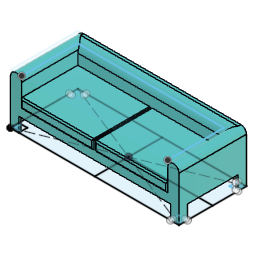
lego_sofa v5 (Autodesk Fusion 360 design; units mm, degrees)
Autodesk Fusion 360 part; units mm, degrees
note: some values were not read from the file. Chosen so that the rebuilt part matches the saved one: which pieces of a blend or face edit are solid.
sketch "Skizze1" plane through (0, 0, 0) normal (0, 0, 1) x (1, 0, 0)
  line L0 (30, -12) -> (-30, -12)
  line L1 (-30, -12) -> (-30, 12)
  line L2 (-30, 12) -> (30, 12)
  line L3 (30, 12) -> (30, -12)
  line L4 (30, -12) -> (-30, 12) construction
  line L5 (-30, -12) -> (30, 12) construction
  dimension "d1" = 60
  dimension "d2" = 24
  constraint horizontal L0
  constraint perpendicular L0 L1
  constraint parallel L0 L2
  constraint parallel L1 L3
  constraint coincident L4 origin
  constraint coincident L5 origin
  measures "d1" distance of L1.end L2.end
  measures "d2" distance of L0.end L1.end
extrude "Extrusion1" add sketch "Skizze1" along normal blind 18
sketch "Skizze2" plane through (0, 0, 0) normal (0, 0, -1) x (1, 0, 0)
  line L0 (-30, -12) -> (30, -12)
  line L1 (30, -12) -> (30, 12)
  line L2 (30, 12) -> (-30, 12)
  line L3 (-30, 12) -> (-30, -12)
  line L4 (-30, 12) -> (-27, 12)
  line L5 (-27, 12) -> (-27, 9)
  line L6 (-27, 9) -> (-30, 9)
  line L7 (-30, 9) -> (-30, 12)
  line L8 (27, 9) -> (30, 9)
  line L9 (27, 12) -> (27, 9)
  line L10 (27, -9) -> (30, -9)
  line L11 (27, -12) -> (27, -9)
  line L12 (-27, -9) -> (-30, -9)
  line L13 (-27, -12) -> (-27, -9)
  line L14 (-29.25, 9.75) -> (-29.25, 11.25)
  line L15 (-29.25, 11.25) -> (-27.75, 11.25)
  line L16 (-29.25, 9.75) -> (-29.25, 9)
  line L17 (-27.75, 11.25) -> (-27, 11.25)
  line L18 (0, 12) -> (0, -12)
  line L19 (0, 0) -> (30, 0)
  line L20 (-29.25, 11.25) -> (-29.25, 9)
  line L21 (-29.25, 11.25) -> (-27, 11.25)
  line L22 (29.25, 11.25) -> (29.25, 9)
  line L23 (29.25, 11.25) -> (27, 11.25)
  line L24 (29.25, -11.25) -> (27, -11.25)
  line L25 (29.25, -11.25) -> (29.25, -9)
  line L26 (-29.25, -11.25) -> (-27, -11.25)
  line L27 (-29.25, -11.25) -> (-29.25, -9)
  dimension "d5" = 3
  dimension "d6" = 3
  constraint horizontal L4
  constraint vertical L5
  constraint horizontal L6
  constraint vertical L7
  constraint coincident L2.end L3.start
  constraint coincident L6 L16.end
  constraint perpendicular L6 L16
  constraint coincident L5 L17.end
  constraint perpendicular L5 L17
  constraint parallel L7 L14
  constraint parallel L4 L15
  constraint midpoint L2 L18.start
  constraint midpoint L0 L18.end
  constraint midpoint L18 L19.start
  constraint midpoint L1 L19.end
  constraint symmetric L14.end L18 L22.start
  constraint symmetric L16.end L18 L22.end
  constraint symmetric L17.end L18 L23.end
  constraint symmetric L19 L22.start L24.start
  constraint symmetric L19 L22.end L25.end
  constraint symmetric L19 L23.end L24.end
  constraint symmetric L18 L24.start L26.start
  constraint symmetric L18 L24.end L26.end
  constraint symmetric L18 L25.end L27.end
  measures "d5" distance of L2.end L4.end
  measures "d6" distance of L2.end L6.end
extrude "Extrusion2" cut sketch "Skizze2" against normal blind 5 contours L0 L2 L3 L5 L6 L12 L13 L18 | L0 L1 L10 L11 L18 L19 | L1 L2 L8 L9 L18 L19
sketch "Skizze3" plane through (0, 0, 18) normal (0, 0, 1) x (-1, 0, 0)
  line L0 (-30, -12) -> (30, -12)
  line L1 (30, -12) -> (30, 12)
  line L2 (30, 12) -> (-30, 12)
  line L3 (-30, 12) -> (-30, -12)
  line L4 (-26, -8) -> (26, -8)
  line L5 (26, -8) -> (26, 8)
  line L6 (-26, 8) -> (-26, -8)
  line L7 (26, 8) -> (26, 12)
  line L8 (-26, 8) -> (-26, 12)
  constraint parallel L0 L4
  constraint parallel L1 L5
  constraint parallel L3 L6
  constraint coincident L2 L7.end
  constraint perpendicular L2 L7
  constraint coincident L2 L8.end
  constraint perpendicular L2 L8
extrude "Extrusion3" cut sketch "Skizze3" against normal blind 7 contours L2 L4 L5 L6 L7 L8
fillet "Abrundung1" radius 3 1 edges at (0, 8, 18)
fillet "Abrundung2" radius 2 4 edges at (30, 0, 18) (26, -0.5, 18) (-26, -0.5, 18) (-30, 0, 18)
extrude "Extrusion4" cut sketch "Skizze2" against normal blind 5 contours L12 L13 L26 L27 | L5 L6 L14 L15 L16 L17 L20 L21 | L10 L11 L24 L25 | L8 L9 L22 L23
sketch "Skizze4" plane through (0, 0, 0) normal (0, 0, -1) x (1, 0, 0)
sketch "Skizze14" plane through (0, 0, 11) normal (0, 0, 1) x (-1, 0, 0)
  line L0 (-26, -8) -> (26, -8)
  line L1 (26, -8) -> (26, 12)
  line L2 (26, 12) -> (-26, 12)
  line L3 (-26, 12) -> (-26, -8)
  line L4 (0.25, -8) -> (0.25, 12)
  line L5 (-0.25, -8) -> (-0.25, 12)
sketch "Skizze15" plane through (0, -12, 0) normal (0, -1, 0) x (1, 0, 0)
  arc A0 (-26, 16) -> (-30, 16) centre (-28, 16) ccw
  line L0 (-30, 16) -> (-30, 0)
  line L1 (-30, 0) -> (-27, 0)
  line L2 (-27, 0) -> (-27, 5)
  line L3 (-27, 5) -> (27, 5)
  line L4 (27, 5) -> (27, 0)
  line L5 (27, 0) -> (30, 0)
  line L6 (30, 0) -> (30, 16)
  arc A1 (30, 16) -> (26, 16) centre (28, 16) ccw
  line L7 (26, 16) -> (26, 11)
  line L8 (26, 11) -> (-26, 11)
  line L9 (-26, 11) -> (-26, 16)
  line L10 (-26, 11) -> (-26, 8)
  line L11 (-26, 8) -> (0, 8)
  line L12 (0, 8) -> (26, 8)
  line L13 (26, 8) -> (26, 11)
  line L14 (0.25, 8) -> (0.25, 11)
  line L15 (-0.25, 8) -> (-0.25, 11)
  dimension "d26" = 3
  dimension "d27" = 26
  constraint coincident L8.end L9.start
  constraint perpendicular L8 L10
  constraint perpendicular L10 L11
  constraint coincident L7.end L8.start
  measures "d26" distance of L8.end L10.end
  measures "d27" distance of L11.end L12.end
extrude "Extrusion6" add sketch "Skizze14" along normal blind 0.3 contours L0 L2 L3 L5 | L0 L1 L2 L4
extrude "Extrusion7" add sketch "Skizze15" along normal blind 0.3 contours L8 L10 L11 L15 | L8 L12 L13 L14
extrude "Extrusion8" add 2 faces at (-17.4167, -12.1, 11) (17.4167, -12.2, 11) along direction (0, 0, 1) blind 0.3
fillet "Abrundung4" radius 0.5 8 edges at (-26, -12.3, 9.65) (-13.125, -12.3, 11.3) (-13.125, -12.3, 8) (-0.25, -12.3, 9.65) (26, -12.3, 9.65) (13.125, -12.3, 11.3) (13.125, -12.3, 8) (0.25, -12.3, 9.65)
fillet "Abrundung5" radius 0.25 4 edges at (-0.3964, -12.1536, 11.1536) (-0.25, -1.9, 11.3) (0.25, -1.9, 11.3) (0.3964, -12.1536, 11.1536)
